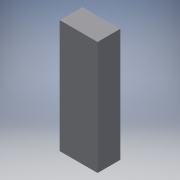
# Autodesk Inventor part: base2_2
Saved by Autodesk Inventor 2019 (Build 230136000, 136)
## iProperties
Created: 2020-03-13
Part Number: base2_2
Material: Generic
Document SubType Name: Modeling
Designer: Pulag
Density: 1 g/cm^3
Appearance: Default
Author: Pulag
Autodesk Inventor part; units mm, degrees
ref_plane "YZ Plane" through (0, 0, 0) normal (1, 0, 0) x (0, 1, 0)
ref_plane "XZ Plane" through (0, 0, 0) normal (0, 1, 0) x (-1, 0, 0)
sketch "Sketch1" plane through (0, 0, 0) normal (0, 0, 1) x (1, 0, 0)
  line L0 (-11.5, -30) -> (-11.5, 20) projected
  line L1 (-11.5, 20) -> (-28.5, 20) projected
  line L2 (-28.5, 20) -> (-28.5, -30) projected
  line L3 (-28.5, -30) -> (-11.5, -30) projected
  line L4 (-8.5, 20) -> (-8.5, -30) projected
  line L5 (-8.5, -30) -> (8.5, -30) projected
  line L6 (8.5, -30) -> (8.5, 20) projected
  line L7 (8.5, 20) -> (-8.5, 20) projected
  line L8 (11.5, 20) -> (11.5, -30) projected
  line L9 (11.5, -30) -> (28.5, -30) projected
  line L10 (28.5, -30) -> (28.5, 20) projected
  line L11 (28.5, 20) -> (11.5, 20) projected
  circle A0 centre (0, 0) radius 8.5 projected
  line L12 (-31, 43.5) -> (-32.5, 43.5) projected
  line L13 (-32.5, 43.5) -> (-32.5, 96.5) projected
  line L14 (-32.5, 96.5) -> (-31, 96.5) projected
  line L15 (-31, 96.5) -> (-31, 43.5) projected
  line L16 (4, 96.5) -> (4, 43.5) projected
  line L17 (4, 43.5) -> (2.5, 43.5) projected
  line L18 (2.5, 43.5) -> (2.5, 96.5) projected
  line L19 (2.5, 96.5) -> (4, 96.5) projected
  line L20 (31, 43.5) -> (31, 96.5) projected
  line L21 (31, 96.5) -> (32.5, 96.5) projected
  line L22 (32.5, 96.5) -> (32.5, 43.5) projected
  line L23 (32.5, 43.5) -> (31, 43.5) projected
  line L24 (-4, 96.5) -> (-2.5, 96.5) projected
  line L25 (-2.5, 96.5) -> (-2.5, 43.5) projected
  line L26 (-2.5, 43.5) -> (-4, 43.5) projected
  line L27 (-4, 43.5) -> (-4, 96.5) projected
  line L28 (-35, 105) -> (-35, -35) projected
  line L29 (-35, -35) -> (35, -35) projected
  line L30 (35, -35) -> (35, 105) projected
  line L31 (35, 105) -> (-35, 105) projected
  line L32 (35, -35) -> (35, -20)
  line L33 (-35, -20) -> (-35, -35)
  line L34 (-35, -35) -> (-30, -35)
  line L35 (-30, -35) -> (-30, -20)
  line L36 (-30, -20) -> (-35, -20)
  line L37 (-35, -20) -> (-35, -35)
  line L38 (35, -35) -> (30, -35)
  line L39 (30, -35) -> (30, -20)
  line L40 (30, -20) -> (35, -20)
  line L41 (35, -20) -> (35, -35)
  line L42 (-35, -35) -> (-30, -35)
  line L43 (30, -35) -> (35, -35)
  point P0 (0, 0)
  dimension "d1" = 5
  dimension "d2" = 15
  dimension "d3" = 5
  dimension "d4" = 15
  constraints: 24 end point, 5 parallel, 4 horizontal, 4 perpendicular
  measures "d1" distance of L33.start L35.end
  measures "d2" distance of L35.end L34.end
  measures "d3" distance of L32.end L39.end
  measures "d4" distance of L38.end L39.end
ref_plane "Work Plane1" through (-35.7285, -35.3642, -3) normal (0, 0, -1) x (0, 1, 0)
extrude "Extrusion1" add sketch "Sketch1" against normal up to surface (3 mm away) contours L36 L35 L29 L28
body "Solid1"
